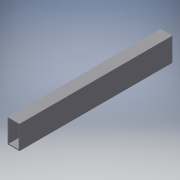
# Autodesk Inventor part: Frame Channle Close
Saved by Autodesk Inventor 2018 (Build 220112000, 112)
## iProperties
Created: 2018-01-22
Part Number: Frame Channle Close
Material: Generic
Document SubType Name: Modeling
Designer: Apple
Density: 1 g/cm^3
Appearance: Default
Author: Apple
Autodesk Inventor part; units mm, degrees
ref_plane "YZ Plane" through (0, 0, 0) normal (1, 0, 0) x (0, 1, 0)
ref_plane "XZ Plane" through (0, 0, 0) normal (0, 1, 0) x (-1, 0, 0)
ref_plane "XY Plane" through (0, 0, 0) normal (0, 0, 1) x (1, 0, 0)
sketch "Sketch1" plane through (0, 0, 0) normal (0, 0, 1) x (1, 0, 0)
  line L0 (23.4477, 29.3492) -> (-14.6523, 29.3492)
  line L1 (-14.6523, 29.3492) -> (-14.6523, -46.8508)
  line L2 (-14.6523, -46.8508) -> (23.4477, -46.8508)
  line L3 (23.4477, -46.8508) -> (23.4477, 29.3492)
  line L4 (20.2727, 26.1742) -> (-11.4773, 26.1742)
  line L5 (-11.4773, 26.1742) -> (-11.4773, -43.6758)
  line L6 (-11.4773, -43.6758) -> (20.2727, -43.6758)
  line L7 (20.2727, -43.6758) -> (20.2727, 26.1742)
  point P0 (0, 0)
  dimension "d0" = 76.2
  dimension "d1" = 38.1
  dimension "d2" = 3.175
  constraints: 16 end point, 4 parallel, 2 perpendicular, 1 horizontal, 3 other
  measures "d0" distance of L2.end L0.start
  measures "d1" distance of L1.end L2.end
  measures "d2" distance between parallel lines of L3 L7
extrude "Extrusion1" add sketch "Sketch1" along normal blind 460.375
body "Solid1"
